Autodesk Fusion 360 part; units mm, degrees
note: some values were not read from the file. Set by a fixed rule: which sketch regions a step uses.
(part 3 of 4)
sketch "Boceto2" plane through (0, 0, 0) normal (0, 0, 1) x (1, 0, 0)
  line L0 (0, 0) -> (609.6, 0)
  line L1 (609.6, 0) -> (609.6, 800)
  line L2 (609.6, 800) -> (0, 800)
  line L3 (0, 800) -> (0, 0)
  line L4 (50, 750) -> (50, 50)
  line L5 (50, 50) -> (559.6, 50)
  line L6 (559.6, 50) -> (559.6, 750)
  line L7 (559.6, 750) -> (50, 750)
  line L8 (-347.6805, -725) -> (-296.8805, -725)
  line L9 (-347.6805, -725) -> (-296.8805, -725)
  line L10 (-525, -725) -> (-347.6805, -725)
  line L11 (-347.6805, -725) -> (-296.8805, -725)
  line L12 (-525, -725) -> (-347.6805, -725)
  line L13 (-347.6805, -725) -> (-373.0805, -725)
  line L14 (-525, -725) -> (-347.6805, -725)
  circle A0 centre (-525, -725) radius 228.1195
  line L15 (-347.6805, -725) -> (-373.0805, -725)
  circle A1 centre (-525, -725) radius 228.1195
  circle A2 centre (-373.0805, -725) radius 2.1
  line L16 (-347.6805, -725) -> (-296.8805, -725)
  circle A3 centre (-525, -725) radius 228.1195
  line L17 (-347.6805, -725) -> (-355.9463, -725)
  line L18 (-525, -725) -> (-525, -547.6805)
  line L19 (-525, -725) -> (-525, -547.6805)
  line L20 (-347.6805, -725) -> (-373.0805, -725)
  line L21 (-347.6805, -725) -> (-355.9463, -725)
  line L22 (-347.6805, -725) -> (-355.9463, -725)
  line L23 (-525, -725) -> (-525, -547.6805)
  line L24 (-525, -725) -> (-525, -547.6805)
  line L25 (-347.6805, -725) -> (-355.9463, -725)
  line L26 (-525, -725) -> (-347.6805, -725)
  line L27 (-525, -725) -> (-347.6805, -725)
  line L28 (-525, -725) -> (-347.6805, -725)
  line L29 (-347.6805, -725) -> (-355.9463, -725)
  line L30 (-347.6805, -725) -> (-296.8805, -725)
  line L31 (-347.6805, -725) -> (-296.8805, -725)
  line L32 (-347.6805, -725) -> (-355.9463, -725)
  line L33 (-347.6805, -725) -> (-296.8805, -725)
  line L34 (-347.6805, -725) -> (-296.8805, -725)
  line L35 (-525, -725) -> (-347.6805, -725)
  line L36 (-347.6805, -725) -> (-355.9463, -725)
  line L37 (-347.6805, -725) -> (-355.9463, -725)
  line L38 (-347.6805, -725) -> (-296.8805, -725)
  line L39 (-347.6805, -725) -> (-355.9463, -725)
  line L40 (-347.6805, -725) -> (-296.8805, -725)
  line L41 (-347.6805, -725) -> (-296.8805, -725)
  line L42 (-525, -725) -> (-347.6805, -725)
  line L43 (-347.6805, -725) -> (-373.0805, -725)
  line L44 (-347.6805, -725) -> (-373.0805, -725)
  line L45 (-525, -725) -> (-525, -547.6805)
  line L46 (-525, -725) -> (-525, -547.6805)
  line L47 (-347.6805, -725) -> (-373.0805, -725)
  circle A4 centre (-525, -725) radius 228.1195
  line L48 (-347.6805, -725) -> (-373.0805, -725)
  line L49 (-347.6805, -725) -> (-373.0805, -725)
  line L50 (-347.6805, -725) -> (-296.8805, -725)
  line L51 (-525, -725) -> (-525, -547.6805)
  line L52 (-347.6805, -725) -> (-373.0805, -725)
  line L53 (-347.6805, -725) -> (-296.8805, -725)
  circle A5 centre (-525, -725) radius 228.1195
  line L54 (-525, -725) -> (-525, -547.6805)
  line L55 (-347.6805, -725) -> (-355.9463, -725)
  line L56 (-347.6805, -725) -> (-355.9463, -725)
  line L57 (-525, -725) -> (-525, -547.6805)
  line L58 (-347.6805, -725) -> (-373.0805, -725)
  line L59 (-525, -725) -> (-525, -547.6805)
  line L60 (-347.6805, -725) -> (-355.9463, -725)
  line L61 (-347.6805, -725) -> (-355.9463, -725)
  line L62 (-525, -725) -> (-525, -547.6805)
  line L63 (-525, -725) -> (-347.6805, -725)
  line L64 (-525, -725) -> (-347.6805, -725)
  line L65 (-525, -725) -> (-347.6805, -725)
  line L66 (-525, -725) -> (-347.6805, -725)
  line L67 (-347.6805, -725) -> (-296.8805, -725)
  line L68 (-347.6805, -725) -> (-355.9463, -725)
  line L69 (-525, -725) -> (-347.6805, -725)
  line L70 (-347.6805, -725) -> (-296.8805, -725)
  line L71 (-347.6805, -725) -> (-355.9463, -725)
  circle A6 centre (-525, -725) radius 228.1195
  circle A7 centre (-525, -725) radius 228.1195
  circle A8 centre (-525, -725) radius 228.1195
  circle A9 centre (-525, -725) radius 228.1195
  line L72 (-525, -725) -> (-347.6805, -725)
  line L73 (-347.6805, -725) -> (-373.0805, -725)
  line L74 (-347.6805, -725) -> (-373.0805, -725)
  line L75 (-347.6805, -725) -> (-373.0805, -725)
  circle A10 centre (-525, -725) radius 228.1195
  line L76 (-347.6805, -725) -> (-373.0805, -725)
  circle A11 centre (-525, -725) radius 228.1195
  line L77 (-347.6805, -725) -> (-373.0805, -725)
  line L78 (-525, -725) -> (-347.6805, -725)
  circle A12 centre (-525, -725) radius 228.1195
  circle A13 centre (-373.0805, -725) radius 2.1
  circle A14 centre (-373.0805, -725) radius 2.1
  circle A15 centre (-373.0805, -725) radius 2.1
  line L79 (-347.6805, -725) -> (-373.0805, -725)
  line L80 (-347.6805, -725) -> (-355.9463, -725)
  line L81 (-525, -725) -> (-347.6805, -725)
  circle A16 centre (-525, -725) radius 228.1195
  circle A17 centre (-525, -725) radius 228.1195
  line L82 (-347.6805, -725) -> (-296.8805, -725)
  circle A18 centre (-525, -725) radius 228.1195
  line L83 (-525, -547.6805) -> (-525, -573.0805)
  circle A19 centre (-525, -573.0805) radius 2.1
  line L84 (-525, -547.6805) -> (-525, -573.0805)
  circle A20 centre (-525, -573.0805) radius 2.1
  line L85 (-525, -547.6805) -> (-525, -573.0805)
  line L86 (-525, -547.6805) -> (-525, -573.0805)
  line L87 (-525, -725) -> (-525, -547.6805)
  circle A21 centre (-525, -573.0805) radius 2.1
  line L88 (-525, -547.6805) -> (-525, -573.0805)
  line L89 (-525, -547.6805) -> (-525, -573.0805)
  line L90 (-525, -902.3195) -> (-525, -876.9195)
  line L91 (-525, -725) -> (-702.3195, -725)
  line L92 (-525, -725) -> (-702.3195, -725)
  line L93 (-525, -902.3195) -> (-525, -876.9195)
  line L94 (-525, -725) -> (-525, -547.6805)
  circle A22 centre (-525, -876.9195) radius 2.1
  circle A23 centre (-525, -573.0805) radius 2.1
  circle A24 centre (-525, -573.0805) radius 2.1
  line L95 (-525, -547.6805) -> (-525, -573.0805)
  line L96 (-525, -902.3195) -> (-525, -876.9195)
  line L97 (-525, -547.6805) -> (-525, -573.0805)
  line L98 (-525, -547.6805) -> (-525, -573.0805)
  circle A25 centre (-525, -573.0805) radius 2.1
  line L99 (-525, -725) -> (-702.3195, -725)
  line L100 (-525, -725) -> (-702.3195, -725)
  line L101 (-525, -547.6805) -> (-525, -573.0805)
  line L102 (-525, -725) -> (-702.3195, -725)
  circle A26 centre (-525, -573.0805) radius 2.1
  line L103 (-525, -547.6805) -> (-525, -573.0805)
  line L104 (-525, -547.6805) -> (-525, -573.0805)
  line L105 (-525, -725) -> (-525, -902.3195)
  circle A27 centre (-525, -876.9195) radius 2.1
  line L106 (-525, -725) -> (-525, -902.3195)
  line L107 (-525, -547.6805) -> (-525, -573.0805)
  circle A28 centre (-525, -876.9195) radius 2.1
  line L108 (-525, -902.3195) -> (-525, -876.9195)
  circle A29 centre (-525, -573.0805) radius 2.1
  circle A30 centre (-525, -573.0805) radius 2.1
  line L109 (-525, -725) -> (-525, -547.6805)
  line L110 (-525, -725) -> (-525, -547.6805)
  circle A31 centre (-525, -876.9195) radius 2.1
  circle A32 centre (-525, -573.0805) radius 2.1
  line L111 (-525, -902.3195) -> (-525, -876.9195)
  line L112 (-525, -725) -> (-525, -902.3195)
  line L113 (-525, -725) -> (-525, -902.3195)
  line L114 (-525, -902.3195) -> (-525, -876.9195)
  line L115 (-525, -725) -> (-525, -902.3195)
  line L116 (-525, -725) -> (-525, -547.6805)
  line L117 (-525, -547.6805) -> (-525, -573.0805)
  line L118 (-525, -725) -> (-702.3195, -725)
  line L119 (-525, -725) -> (-702.3195, -725)
  circle A33 centre (-525, -573.0805) radius 2.1
  line L120 (-525, -902.3195) -> (-525, -876.9195)
  line L121 (-525, -547.6805) -> (-525, -573.0805)
  circle A34 centre (-525, -573.0805) radius 2.1
  circle A35 centre (-525, -573.0805) radius 2.1
  line L122 (-525, -902.3195) -> (-525, -876.9195)
  line L123 (-525, -725) -> (-525, -902.3195)
  circle A36 centre (-525, -573.0805) radius 2.1
  line L124 (-525, -547.6805) -> (-525, -573.0805)
  line L125 (-525, -725) -> (-702.3195, -725)
  circle A37 centre (-525, -573.0805) radius 2.1
  circle A38 centre (-525, -573.0805) radius 2.1
  circle A39 centre (-525, -876.9195) radius 2.1
  circle A40 centre (-676.9195, -725) radius 2.1
  line L126 (-525, -725) -> (-702.3195, -725)
  circle A41 centre (-676.9195, -725) radius 2.1
  circle A42 centre (-676.9195, -725) radius 2.1
  line L127 (-702.3195, -725) -> (-676.9195, -725)
  line L128 (-525, -902.3195) -> (-525, -876.9195)
  circle A43 centre (-676.9195, -725) radius 2.1
  circle A44 centre (-676.9195, -725) radius 2.1
  line L129 (-525, -902.3195) -> (-525, -876.9195)
  line L130 (-525, -725) -> (-525, -902.3195)
  circle A45 centre (-525, -876.9195) radius 2.1
  line L131 (-525, -725) -> (-702.3195, -725)
  circle A46 centre (-525, -876.9195) radius 2.1
  line L132 (-525, -725) -> (-525, -902.3195)
  line L133 (-525, -725) -> (-525, -902.3195)
  line L134 (-525, -725) -> (-525, -902.3195)
  circle A47 centre (-525, -876.9195) radius 2.1
  line L135 (-525, -725) -> (-702.3195, -725)
  line L136 (-525, -725) -> (-702.3195, -725)
  line L137 (-702.3195, -725) -> (-676.9195, -725)
  line L138 (-702.3195, -725) -> (-676.9195, -725)
  circle A48 centre (-676.9195, -725) radius 2.1
  line L139 (-525, -902.3195) -> (-525, -876.9195)
  circle A49 centre (-525, -876.9195) radius 2.1
  line L140 (-525, -725) -> (-525, -902.3195)
  line L141 (-525, -725) -> (-525, -902.3195)
  circle A50 centre (-525, -876.9195) radius 2.1
  circle A51 centre (-525, -876.9195) radius 2.1
  line L142 (-525, -725) -> (-702.3195, -725)
  line L143 (-525, -902.3195) -> (-525, -876.9195)
  line L144 (-525, -725) -> (-702.3195, -725)
  line L145 (-525, -725) -> (-702.3195, -725)
  line L146 (-525, -902.3195) -> (-525, -876.9195)
  circle A52 centre (-525, -876.9195) radius 2.1
  circle A53 centre (-525, -876.9195) radius 2.1
  line L147 (-525, -725) -> (-525, -902.3195)
  line L148 (-525, -902.3195) -> (-525, -876.9195)
  line L149 (-525, -902.3195) -> (-525, -876.9195)
  circle A54 centre (-676.9195, -725) radius 2.1
  line L150 (-525, -725) -> (-525, -902.3195)
  circle A55 centre (-676.9195, -725) radius 2.1
  line L151 (-525, -725) -> (-702.3195, -725)
  line L152 (-525, -902.3195) -> (-525, -876.9195)
  circle A56 centre (-676.9195, -725) radius 2.1
  line L153 (-525, -725) -> (-525, -902.3195)
  line L154 (-525, -725) -> (-525, -902.3195)
  circle A57 centre (-525, -876.9195) radius 2.1
  circle A58 centre (-525, -876.9195) radius 2.1
  circle A59 centre (-525, -876.9195) radius 2.1
  circle A60 centre (-676.9195, -725) radius 2.1
  line L155 (-702.3195, -725) -> (-676.9195, -725)
  line L156 (-702.3195, -725) -> (-676.9195, -725)
  line L157 (-702.3195, -725) -> (-676.9195, -725)
  line L158 (-702.3195, -725) -> (-676.9195, -725)
  line L159 (-702.3195, -725) -> (-676.9195, -725)
  circle A61 centre (-676.9195, -725) radius 2.1
  line L160 (-702.3195, -725) -> (-676.9195, -725)
  line L161 (-702.3195, -725) -> (-676.9195, -725)
  circle A62 centre (-676.9195, -725) radius 2.1
  line L162 (-702.3195, -725) -> (-676.9195, -725)
  line L163 (-702.3195, -725) -> (-676.9195, -725)
  circle A63 centre (-676.9195, -725) radius 2.1
  circle A64 centre (-676.9195, -725) radius 2.1
  line L164 (-702.3195, -725) -> (-676.9195, -725)
  line L165 (-702.3195, -725) -> (-676.9195, -725)
  line L166 (-702.3195, -725) -> (-676.9195, -725)
  circle A65 centre (-676.9195, -725) radius 2.1
  circle A66 centre (-676.9195, -725) radius 2.1
  line L167 (-702.3195, -725) -> (-676.9195, -725)
  circle A67 centre (-373.0805, -725) radius 2.1
  circle A68 centre (-373.0805, -725) radius 2.1
  circle A69 centre (-373.0805, -725) radius 2.1
  circle A70 centre (-525, -725) radius 228.1195
  circle A71 centre (-373.0805, -725) radius 2.1
  circle A72 centre (-373.0805, -725) radius 2.1
  circle A73 centre (-373.0805, -725) radius 2.1
  circle A74 centre (-373.0805, -725) radius 2.1
  circle A75 centre (-373.0805, -725) radius 2.1
  circle A76 centre (-373.0805, -725) radius 2.1
  circle A77 centre (-373.0805, -725) radius 2.1
  circle A78 centre (-373.0805, -725) radius 2.1
  circle A79 centre (-373.0805, -725) radius 2.1
  circle A80 centre (-525, -725) radius 228.1195
  circle A81 centre (304.8, 400) radius 228.1195
  circle A82 centre (304.8, 400) radius 238.1195
  dimension "d627" = 609.6
  dimension "d628" = 800
  dimension "d736" = -50
  dimension "d737" = 177.3195
  dimension "d738" = 177.3195
  dimension "d739" = 177.3195
  dimension "d740" = 177.3195
  dimension "d741" = 25.4
  dimension "d742" = 25.4
  dimension "d743" = 25.4
  dimension "d744" = 25.4
  dimension "d745" = 4.2
  dimension "d746" = 4.2
  dimension "d747" = 4.2
  dimension "d748" = 4.2
  dimension "d749" = 50.8
  dimension "d750" = 177.3195
  dimension "d751" = 177.3195
  dimension "d752" = 177.3195
  dimension "d753" = 177.3195
  dimension "d754" = 25.4
  dimension "d755" = 25.4
  dimension "d756" = 25.4
  dimension "d757" = 25.4
  dimension "d758" = 4.2
  dimension "d759" = 4.2
  dimension "d760" = 4.2
  dimension "d761" = 4.2
  dimension "d762" = 50.8
  dimension "d763" = 177.3195
  dimension "d764" = 177.3195
  dimension "d765" = 177.3195
  dimension "d766" = 177.3195
  dimension "d767" = 25.4
  dimension "d768" = 25.4
  dimension "d769" = 25.4
  dimension "d770" = 25.4
  dimension "d771" = 4.2
  dimension "d772" = 4.2
  dimension "d773" = 4.2
  dimension "d774" = 4.2
  dimension "d775" = 50.8
  dimension "d776" = 177.3195
  dimension "d777" = 177.3195
  dimension "d778" = 177.3195
  dimension "d779" = 177.3195
  dimension "d780" = 25.4
  dimension "d781" = 25.4
  dimension "d782" = 25.4
  dimension "d783" = 25.4
  dimension "d784" = 4.2
  dimension "d785" = 4.2
  dimension "d786" = 4.2
  dimension "d787" = 4.2
  dimension "d788" = 50.8
  dimension "d789" = 177.3195
  dimension "d790" = 177.3195
  dimension "d791" = 177.3195
  dimension "d792" = 177.3195
  dimension "d793" = 25.4
  dimension "d794" = 25.4
  dimension "d795" = 25.4
  dimension "d796" = 25.4
  dimension "d797" = 4.2
  dimension "d798" = 4.2
  dimension "d799" = 4.2
  dimension "d800" = 4.2
  dimension "d801" = 50.8
  dimension "d802" = 177.3195
  dimension "d803" = 177.3195
  dimension "d804" = 177.3195
  dimension "d805" = 177.3195
  dimension "d806" = 25.4
  dimension "d807" = 25.4
  dimension "d808" = 25.4
  dimension "d809" = 25.4
  dimension "d810" = 4.2
  dimension "d811" = 4.2
  dimension "d812" = 4.2
  dimension "d813" = 4.2
  dimension "d814" = 50.8
  dimension "d815" = 177.3195
  dimension "d816" = 177.3195
  dimension "d817" = 177.3195
  dimension "d818" = 177.3195
  dimension "d819" = 25.4
  dimension "d820" = 25.4
  dimension "d821" = 25.4
  dimension "d822" = 25.4
  dimension "d823" = 4.2
  dimension "d824" = 4.2
  dimension "d825" = 4.2
  dimension "d826" = 4.2
  dimension "d827" = 50.8
  dimension "d828" = 177.3195
  dimension "d829" = 177.3195
  dimension "d830" = 177.3195
  dimension "d831" = 177.3195
  dimension "d832" = 25.4
  dimension "d833" = 25.4
  dimension "d834" = 25.4
  dimension "d835" = 25.4
  dimension "d836" = 4.2
  dimension "d837" = 4.2
  dimension "d838" = 4.2
  dimension "d839" = 4.2
  dimension "d840" = 50.8
  dimension "d841" = 177.3195
  dimension "d842" = 177.3195
  dimension "d843" = 177.3195
  dimension "d844" = 177.3195
  dimension "d845" = 25.4
  dimension "d846" = 25.4
  dimension "d847" = 25.4
  dimension "d848" = 25.4
  dimension "d849" = 4.2
  dimension "d850" = 4.2
  dimension "d851" = 4.2
  dimension "d852" = 4.2
  dimension "d853" = 50.8
  dimension "d854" = 177.3195
  dimension "d855" = 177.3195
  dimension "d856" = 177.3195
  dimension "d857" = 177.3195
  dimension "d858" = 25.4
  dimension "d859" = 25.4
  dimension "d860" = 25.4
  dimension "d861" = 25.4
  dimension "d862" = 4.2
  dimension "d863" = 4.2
  dimension "d864" = 4.2
  dimension "d865" = 4.2
  dimension "d866" = 50.8
  dimension "d867" = 177.3195
  dimension "d868" = 177.3195
  dimension "d869" = 177.3195
  dimension "d870" = 177.3195
  dimension "d871" = 25.4
  dimension "d872" = 25.4
  dimension "d873" = 25.4
  dimension "d874" = 25.4
  dimension "d875" = 4.2
  dimension "d876" = 4.2
  dimension "d877" = 4.2
  dimension "d878" = 4.2
  dimension "d879" = 50.8
  dimension "d880" = 177.3195
  dimension "d881" = 177.3195
  dimension "d882" = 177.3195
  dimension "d883" = 177.3195
  dimension "d884" = 25.4
  dimension "d885" = 25.4
  dimension "d886" = 25.4
  dimension "d887" = 25.4
  dimension "d888" = 4.2
  dimension "d889" = 4.2
  dimension "d890" = 4.2
  dimension "d891" = 4.2
  dimension "d892" = 50.8
  dimension "d893" = 177.3195
  dimension "d894" = 177.3195
  dimension "d895" = 177.3195
  dimension "d896" = 177.3195
  dimension "d897" = 25.4
  dimension "d898" = 25.4
  dimension "d904" = 25.4
  dimension "d905" = 25.4
  dimension "d906" = 4.2
  dimension "d912" = 4.2
  dimension "d916" = 4.2
  dimension "d917" = 4.2
  dimension "d918" = 50.8
  dimension "d921" = 177.3195
  dimension "d922" = 177.3195
  dimension "d924" = 177.3195
  dimension "d925" = 177.3195
  dimension "d926" = 25.4
  dimension "d929" = 25.4
  dimension "d930" = 25.4
  dimension "d931" = 25.4
  dimension "d932" = 4.2
  dimension "d934" = 4.2
  dimension "d935" = 4.2
  dimension "d936" = 4.2
  dimension "d940" = 50.8
  dimension "d944" = 177.3195
  dimension "d945" = 177.3195
  dimension "d946" = 177.3195
  dimension "d947" = 177.3195
  dimension "d948" = 25.4
  dimension "d951" = 25.4
  dimension "d952" = 25.4
  dimension "d953" = 25.4
  dimension "d954" = 4.2
  dimension "d955" = 4.2
  dimension "d956" = 4.2
  dimension "d957" = 4.2
  dimension "d958" = 50.8
  dimension "d959" = 177.3195
  dimension "d960" = 177.3195
  dimension "d961" = 177.3195
  dimension "d962" = 177.3195
  dimension "d963" = 25.4
  dimension "d964" = 25.4
  dimension "d965" = 25.4
  dimension "d966" = 25.4
  dimension "d967" = 4.2
  dimension "d968" = 4.2
  dimension "d969" = 4.2
  dimension "d970" = 4.2
  dimension "d971" = 50.8
  dimension "d972" = 456.2391
  dimension "d973" = 456.239
  dimension "d974" = 10
  constraint horizontal L0
  constraint vertical L1
  constraint horizontal L2
  constraint vertical L3
  constraint coincident L0.start L3.end
  constraint vertical L140
  constraint perpendicular L81 L140
  constraint perpendicular L100 L140
  constraint perpendicular L46 L81
  constraint coincident L17.end L81
  constraint parallel L76 L81
  constraint parallel L46 L88
  constraint parallel L100 L157
  constraint parallel L140 L143
  constraint coincident L13.end L15.end
  constraint coincident L83.end A19.centre
  constraint coincident A40.centre A41.centre
  constraint coincident L90.end L93.end
  constraint parallel L70 L81
  constraint coincident L10.start L12.start
  constraint coincident L8.end A6
  constraint vertical L123
  constraint perpendicular L78 L123
  constraint perpendicular L119 L123
  constraint perpendicular L78 L116
  constraint coincident L17.end L78
  constraint parallel L43 L78
  constraint parallel L103 L116
  constraint parallel L119 L160
  constraint parallel L123 L149
  constraint parallel L11 L78
  constraint coincident L8.end A0
  constraint vertical L106
  constraint perpendicular L10 L106
  constraint perpendicular L91 L106
  constraint perpendicular L10 L24
  constraint coincident L17.end L10
  constraint parallel L10 L48
  constraint parallel L24 L101
  constraint parallel L91 L158
  constraint parallel L106 L152
  constraint parallel L10 L38
  constraint coincident L8.end A10
  constraint vertical L147
  constraint perpendicular L66 L147
  constraint perpendicular L118 L147
  constraint perpendicular L45 L66
  constraint coincident L17.end L66
  constraint parallel L13 L66
  constraint parallel L45 L83
  constraint parallel L118 L164
  constraint parallel L120 L147
  constraint parallel L53 L66
  constraint coincident L8.end A7
  constraint vertical L154
  constraint perpendicular L63 L154
  constraint perpendicular L136 L154
  constraint perpendicular L18 L63
  constraint coincident L17.end L63
  constraint parallel L49 L63
  constraint parallel L18 L89
  constraint parallel L136 L137
  constraint parallel L111 L154
  constraint parallel L50 L63
  constraint coincident L8.end A1
  constraint vertical L141
  constraint perpendicular L72 L141
  constraint perpendicular L141 L142
  constraint perpendicular L19 L72
  constraint coincident L17.end L72
  constraint parallel L58 L72
  constraint parallel L19 L104
  constraint parallel L142 L162
  constraint parallel L129 L141
  constraint parallel L8 L72
  constraint coincident L8.end A9
  constraint vertical L115
  constraint perpendicular L28 L115
  constraint perpendicular L92 L115
  constraint perpendicular L28 L110
  constraint coincident L17.end L28
  constraint parallel L28 L77
  constraint parallel L85 L110
  constraint parallel L92 L155
  constraint parallel L108 L115
  constraint parallel L28 L40
  constraint coincident L8.end A11
  constraint vertical L153
  constraint perpendicular L65 L153
  constraint perpendicular L144 L153
  constraint perpendicular L62 L65
  constraint coincident L17.end L65
  constraint parallel L20 L65
  constraint parallel L62 L95
  constraint parallel L144 L165
  constraint parallel L96 L153
  constraint parallel L65 L67
  constraint coincident L8.end A4
  constraint vertical L132
  constraint perpendicular L12 L132
  constraint perpendicular L126 L132
  constraint perpendicular L12 L23
  constraint coincident L17.end L12
  constraint parallel L12 L75
  constraint parallel L23 L124
  constraint parallel L126 L163
  constraint parallel L114 L132
  constraint parallel L12 L82
  constraint coincident L8.end A12
  constraint vertical L112
  constraint perpendicular L35 L112
  constraint perpendicular L112 L151
  constraint perpendicular L35 L109
  constraint coincident L17.end L35
  constraint parallel L35 L79
  constraint parallel L109 L117
  constraint parallel L151 L159
  constraint parallel L112 L139
  constraint parallel L16 L35
  constraint coincident L8.end A70
  constraint vertical L113
  constraint perpendicular L64 L113
  constraint perpendicular L113 L125
  constraint perpendicular L64 L87
  constraint coincident L17.end L64
  constraint parallel L64 L74
  constraint parallel L86 L87
  constraint parallel L125 L166
  constraint parallel L113 L148
  constraint parallel L30 L64
  constraint coincident L8.end A5
  constraint vertical L133
  constraint perpendicular L27 L133
  constraint perpendicular L99 L133
  constraint perpendicular L27 L54
  constraint coincident L17.end L27
  constraint parallel L15 L27
  constraint parallel L54 L98
  constraint parallel L99 L127
  constraint parallel L93 L133
  constraint parallel L27 L34
  constraint coincident L8.end A17
  constraint vertical L130
  constraint perpendicular L14 L130
  constraint perpendicular L130 L131
  constraint perpendicular L14 L94
  constraint coincident L17.end L14
  constraint parallel L14 L52
  constraint parallel L84 L94
  constraint parallel L131 L161
  constraint parallel L122 L130
  constraint parallel L9 L14
  constraint coincident L8.end A8
  constraint vertical L105
  constraint perpendicular L42 L105
  constraint perpendicular L102 L105
  constraint perpendicular L42 L59
  constraint coincident L17.end L42
  constraint parallel L42 L47
  constraint parallel L59 L107
  constraint parallel L102 L156
  constraint parallel L105 L146
  constraint parallel L33 L42
  constraint coincident L8.end A16
  constraint vertical L150
  constraint perpendicular L26 L150
  constraint perpendicular L135 L150
  constraint perpendicular L26 L57
  constraint coincident L17.end L26
  constraint parallel L26 L73
  constraint parallel L57 L97
  constraint parallel L135 L138
  constraint parallel L128 L150
  constraint parallel L26 L31
  constraint coincident L8.end A3
  constraint vertical L134
  constraint perpendicular L69 L134
  constraint perpendicular L134 L145
  constraint perpendicular L51 L69
  constraint coincident L17.end L69
  constraint parallel L44 L69
  constraint parallel L51 L121
  constraint parallel L145 L167
  constraint parallel L90 L134
  constraint parallel L41 L69
  constraint coincident L8.end A18
  measures "d627" distance of L0.start L0.end
  measures "d628" distance of L0.start L2.end
  measures "d737" distance of L10.start L90.start
  measures "d738" distance of L10.start L8.start
  measures "d739" distance of L10.start L91.end
  measures "d740" distance of L10.start L18.end
  measures "d741" distance of L8.start L13.end
  measures "d742" distance of L18.end L83.end
  measures "d743" distance of L91.end A40.centre
  measures "d744" distance of L90.end L90.start
  measures "d745" diameter of A13
  measures "d746" diameter of A37
  measures "d747" diameter of A54
  measures "d748" diameter of A51
  measures "d749" distance of L8.start L8.end
  measures "d750" distance of L90.start L10.start
  measures "d751" distance of L10.start L8.start
  measures "d752" distance of L91.end L10.start
  measures "d753" distance of L18.end L10.start
  measures "d754" distance of L13.end L8.start
  measures "d755" distance of L83.end L18.end
  measures "d756" distance of L91.end A40.centre
  measures "d757" distance of L90.start L90.end
  measures "d758" diameter of A71
  measures "d759" diameter of A30
  measures "d760" diameter of A56
  measures "d761" diameter of A31
  measures "d762" distance of L8.end L8.start
  measures "d763" distance of L10.start L90.start
  measures "d764" distance of L10.start L8.start
  measures "d765" distance of L10.start L91.end
  measures "d766" distance of L10.start L18.end
  measures "d767" distance of L8.start L13.end
  measures "d768" distance of L83.end L18.end
  measures "d769" distance of L91.end A40.centre
  measures "d770" distance of L90.end L90.start
  measures "d771" diameter of A79
  measures "d772" diameter of A19
  measures "d773" diameter of A65
  measures "d774" diameter of A50
  measures "d775" distance of L8.end L8.start
  measures "d776" distance of L10.start L90.start
  measures "d777" distance of L10.start L8.start
  measures "d778" distance of L91.end L10.start
  measures "d779" distance of L18.end L10.start
  measures "d780" distance of L13.end L8.start
  measures "d781" distance of L18.end L83.end
  measures "d782" distance of L91.end A40.centre
  measures "d783" distance of L90.end L90.start
  measures "d784" diameter of A14
  measures "d785" diameter of A33
  measures "d786" diameter of A61
  measures "d787" diameter of A22
  measures "d788" distance of L8.end L8.start
  measures "d789" distance of L90.start L10.start
  measures "d790" distance of L8.start L10.start
  measures "d791" distance of L91.end L10.start
  measures "d792" distance of L18.end L10.start
  measures "d793" distance of L13.end L8.start
  measures "d794" distance of L18.end L83.end
  measures "d795" distance of A40.centre L91.end
  measures "d796" distance of L90.start L90.end
  measures "d797" diameter of A67
  measures "d798" diameter of A38
  measures "d799" diameter of A55
  measures "d800" diameter of A46
  measures "d801" distance of L8.start L8.end
  measures "d802" distance of L90.start L10.start
  measures "d803" distance of L8.start L10.start
  measures "d804" distance of L91.end L10.start
  measures "d805" distance of L18.end L10.start
  measures "d806" distance of L13.end L8.start
  measures "d807" distance of L83.end L18.end
  measures "d808" distance of A40.centre L91.end
  measures "d809" distance of L90.end L90.start
  measures "d810" diameter of A72
  measures "d811" diameter of A25
  measures "d812" diameter of A60
  measures "d813" diameter of A47
  measures "d814" distance of L8.end L8.start
  measures "d815" distance of L10.start L90.start
  measures "d816" distance of L10.start L8.start
  measures "d817" distance of L10.start L91.end
  measures "d818" distance of L10.start L18.end
  measures "d819" distance of L13.end L8.start
  measures "d820" distance of L18.end L83.end
  measures "d821" distance of A40.centre L91.end
  measures "d822" distance of L90.start L90.end
  measures "d823" diameter of A15
  measures "d824" diameter of A23
  measures "d825" diameter of A43
  measures "d826" diameter of A58
  measures "d827" distance of L8.end L8.start
  measures "d828" distance of L90.start L10.start
  measures "d829" distance of L8.start L10.start
  measures "d830" distance of L91.end L10.start
  measures "d831" distance of L18.end L10.start
  measures "d832" distance of L8.start L13.end
  measures "d833" distance of L18.end L83.end
  measures "d834" distance of A40.centre L91.end
  measures "d835" distance of L90.start L90.end
  measures "d836" diameter of A69
  measures "d837" diameter of A35
  measures "d838" diameter of A44
  measures "d839" diameter of A39
  measures "d840" distance of L8.start L8.end
  measures "d841" distance of L90.start L10.start
  measures "d842" distance of L10.start L8.start
  measures "d843" distance of L10.start L91.end
  measures "d844" distance of L18.end L10.start
  measures "d845" distance of L13.end L8.start
  measures "d846" distance of L83.end L18.end
  measures "d847" distance of A40.centre L91.end
  measures "d848" distance of L90.start L90.end
  measures "d849" diameter of A77
  measures "d850" diameter of A21
  measures "d851" diameter of A42
  measures "d852" diameter of A45
  measures "d853" distance of L8.end L8.start
  measures "d854" distance of L90.start L10.start
  measures "d855" distance of L10.start L8.start
  measures "d856" distance of L91.end L10.start
  measures "d857" distance of L10.start L18.end
  measures "d858" distance of L13.end L8.start
  measures "d859" distance of L83.end L18.end
  measures "d860" distance of L91.end A40.centre
  measures "d861" distance of L90.start L90.end
  measures "d862" diameter of A2
  measures "d863" diameter of A29
  measures "d864" diameter of A48
  measures "d865" diameter of A59
  measures "d866" distance of L8.end L8.start
  measures "d867" distance of L10.start L90.start
  measures "d868" distance of L10.start L8.start
  measures "d869" distance of L10.start L91.end
  measures "d870" distance of L10.start L18.end
  measures "d871" distance of L8.start L13.end
  measures "d872" distance of L18.end L83.end
  measures "d873" distance of A40.centre L91.end
  measures "d874" distance of L90.end L90.start
  measures "d875" diameter of A78
  measures "d876" diameter of A24
  measures "d877" diameter of A40
  measures "d878" diameter of A57
  measures "d879" distance of L8.end L8.start
  measures "d880" distance of L10.start L90.start
  measures "d881" distance of L10.start L8.start
  measures "d882" distance of L91.end L10.start
  measures "d883" distance of L18.end L10.start
  measures "d884" distance of L13.end L8.start
  measures "d885" distance of L18.end L83.end
  measures "d886" distance of L91.end A40.centre
  measures "d887" distance of L90.end L90.start
  measures "d888" diameter of A76
  measures "d889" diameter of A36
  measures "d890" diameter of A66
  measures "d891" diameter of A49
  measures "d892" distance of L8.end L8.start
  measures "d893" distance of L90.start L10.start
  measures "d894" distance of L10.start L8.start
  measures "d895" distance of L10.start L91.end
  measures "d896" distance of L18.end L10.start
  measures "d897" distance of L8.start L13.end
  measures "d898" distance of L18.end L83.end
  measures "d904" distance of L91.end A40.centre
  measures "d905" distance of L90.start L90.end
  measures "d906" diameter of A73
  measures "d912" diameter of A20
  measures "d916" diameter of A64
  measures "d917" diameter of A27
  measures "d918" distance of L8.end L8.start
  measures "d921" distance of L10.start L90.start
  measures "d922" distance of L10.start L8.start
  measures "d924" distance of L91.end L10.start
  measures "d925" distance of L18.end L10.start
  measures "d926" distance of L8.start L13.end
  measures "d929" distance of L18.end L83.end
  measures "d930" distance of L91.end A40.centre
  measures "d931" distance of L90.end L90.start
  measures "d932" diameter of A74
  measures "d934" diameter of A26
  measures "d935" diameter of A41
  measures "d936" diameter of A28
  measures "d940" distance of L8.start L8.end
  measures "d944" distance of L10.start L90.start
  measures "d945" distance of L8.start L10.start
  measures "d946" distance of L91.end L10.start
  measures "d947" distance of L10.start L18.end
  measures "d948" distance of L8.start L13.end
  measures "d951" distance of L18.end L83.end
  measures "d952" distance of A40.centre L91.end
  measures "d953" distance of L90.end L90.start
  measures "d954" diameter of A75
  measures "d955" diameter of A34
  measures "d956" diameter of A62
  measures "d957" diameter of A52
  measures "d958" distance of L8.start L8.end
  measures "d959" distance of L10.start L90.start
  measures "d960" distance of L10.start L8.start
  measures "d961" distance of L10.start L91.end
  measures "d962" distance of L10.start L18.end
  measures "d963" distance of L13.end L8.start
  measures "d964" distance of L18.end L83.end
  measures "d965" distance of L91.end A40.centre
  measures "d966" distance of L90.end L90.start
  measures "d967" diameter of A68
  measures "d968" diameter of A32
  measures "d969" diameter of A63
  measures "d970" diameter of A53
  measures "d971" distance of L8.end L8.start
  measures "d972" diameter of A80
  measures "d973" diameter of A81
extrude "Extruir1" add sketch "Boceto2" along normal blind 105 contours L0 L1 L2 L3
extrude "Extruir2" add sketch "Boceto2" along normal blind 50 contours L4 L5 L6 L7 | A81 | A82
sketch "Boceto3" plane through (0, 0, 50) normal (0, 0, 1) x (-1, 0, 0)
  line L0 (-559.6, -750) -> (-50, -750)
  line L1 (-50, -750) -> (-50, -50)
  line L2 (-50, -50) -> (-559.6, -50)
  line L3 (-559.6, -50) -> (-559.6, -750)
  line L4 (-50, -750) -> (-559.6, -750)
  line L5 (-559.6, -750) -> (-559.6, -50)
  line L6 (-50, -50) -> (-50, -750)
  line L7 (-559.6, -50) -> (-50, -50)
  circle A0 centre (-304.8, -400) radius 228.1195
  dimension "d984" = 456.239
  measures "d984" diameter of A0
extrude "Extruir4" add sketch "Boceto3" along normal blind 16
sketch "Boceto4" plane through (0, 0, 66) normal (0, 0, 1) x (-1, 0, 0)
  circle A0 centre (-304.8, -400) radius 228.1195
  line L0 (-559.6, -50) -> (-559.6, -750)
  line L1 (-559.6, -750) -> (-50, -750)
  line L2 (-50, -750) -> (-50, -50)
  line L3 (-50, -50) -> (-559.6, -50)
  circle A1 centre (-304.8, -400) radius 228.1195
  circle A2 centre (-304.8, -400) radius 228.1195
  circle A3 centre (-304.8, -400) radius 238.1195
  dimension "d987" = 10
  constraint concentric A1 A2
extrude "Extruir5" add sketch "Boceto4" along normal blind 20 contours L0 L1 L2 L3
fillet "Empalme1" radius 225 1 edges at (526.8053, 486.1077, 66)
sketch "Boceto5" plane through (609.6, 0, 0) normal (1, 0, 0) x (0, 1, 0)
  line L0 (0, 0) -> (800, 0)
  line L1 (800, 0) -> (800, 105)
  line L2 (800, 105) -> (0, 105)
  line L3 (0, 105) -> (0, 0)
  line L4 (0, 105) -> (800, 105)
  line L5 (0, 0) -> (0, 105)
  line L6 (0, 0) -> (800, 0)
  line L7 (800, 0) -> (800, 105)
  line L8 (0, 0) -> (800, 0)
  line L9 (800, 0) -> (800, 50)
  line L10 (800, 50) -> (0, 50)
  line L11 (0, 50) -> (0, 0)
  line L12 (0, 50) -> (0, 25)
  line L13 (0, 50) -> (100, 50)
  line L14 (0, 15) -> (0, 50)
  line L15 (0, 0) -> (140, 0)
  line L16 (140, 0) -> (140, 25)
  line L17 (140, 25) -> (0, 25)
  line L18 (0, 25) -> (0, 0)
  line L19 (140, 25) -> (140, 35)
  line L20 (140, 35) -> (300, 35)
  line L21 (300, 35) -> (300, 15)
  line L22 (300, 15) -> (140, 15)
  line L23 (140, 15) -> (140, 35)
  line L24 (800, 50) -> (660, 50)
  line L25 (660, 50) -> (660, 25)
  line L26 (660, 25) -> (800, 25)
  line L27 (800, 25) -> (800, 50)
  line L28 (660, 25) -> (660, 35)
  line L29 (660, 35) -> (500, 35)
  line L30 (500, 35) -> (500, 15)
  line L31 (500, 15) -> (660, 15)
  line L32 (660, 15) -> (660, 35)
  line L33 (300, 25) -> (500, 25)
  circle A0 centre (400, 25) radius 10
  circle A1 centre (400, 25) radius 19
  line L34 (659, 44) -> (501, 44)
  line L35 (491, 34) -> (491, 16)
  line L36 (501, 6) -> (659, 6)
  line L37 (669, 16) -> (669, 34)
  line L38 (143, 42) -> (297, 42)
  line L39 (307, 32) -> (307, 18)
  line L40 (297, 8) -> (143, 8)
  line L41 (133, 18) -> (133, 32)
  arc A2 (143, 42) -> (133, 32) centre (143, 32) ccw
  arc A3 (133, 18) -> (143, 8) centre (143, 18) ccw
  arc A4 (307, 32) -> (297, 42) centre (297, 32) ccw
  arc A5 (297, 8) -> (307, 18) centre (297, 18) ccw
  arc A6 (501, 44) -> (491, 34) centre (501, 34) ccw
  arc A7 (491, 16) -> (501, 6) centre (501, 16) ccw
  arc A8 (659, 6) -> (669, 16) centre (659, 16) ccw
  arc A9 (669, 34) -> (659, 44) centre (659, 34) ccw
  dimension "d992" = 800
  dimension "d993" = 50
  dimension "d997" = 140
  dimension "d998" = 10
  dimension "d999" = 160
  dimension "d1000" = 20
  dimension "d1001" = 140
  dimension "d1002" = 10
  dimension "d1003" = 160
  dimension "d1004" = 20
  dimension "d1005" = 9
  dimension "d1008" = 10
  dimension "d1009" = 10
  constraint horizontal L8
  constraint vertical L9
  constraint horizontal L10
  constraint vertical L11
  constraint coincident L0.start L3.end
  constraint midpoint L11 L12.end
  constraint horizontal L13
  constraint vertical L14
  constraint horizontal L15
  constraint vertical L16
  constraint horizontal L17
  constraint vertical L18
  constraint perpendicular L10 L19
  constraint horizontal L20
  constraint vertical L21
  constraint horizontal L22
  constraint vertical L23
  constraint horizontal L24
  constraint vertical L25
  constraint horizontal L26
  constraint vertical L27
  constraint perpendicular L26 L28
  constraint horizontal L29
  constraint vertical L30
  constraint horizontal L31
  constraint vertical L32
  constraint midpoint L21 L33.start
  constraint midpoint L30 L33.end
  constraint perpendicular L30 L33
  constraint midpoint L33 A0.centre
  constraint tangent L38 A2
  constraint tangent L41 A2
  constraint tangent L40 A3
  constraint tangent L41 A3
  constraint equal A2 A3
  constraint tangent L38 A4
  constraint tangent L39 A4
  constraint tangent L39 A5
  constraint tangent L40 A5
  constraint equal A4 A5
  constraint tangent L34 A6
  constraint tangent L35 A6
  constraint equal A4 A6
  constraint tangent L36 A7
  constraint tangent L35 A7
  constraint equal A4 A7
  constraint tangent L36 A8
  constraint tangent L37 A8
  constraint equal A4 A8
  constraint tangent L34 A9
  constraint tangent L37 A9
  constraint equal A4 A9
  measures "d992" distance of L0.start L0.end
  measures "d993" distance of L0.start L10.end
  measures "d997" distance of L0.start L15.end
  measures "d998" distance of L16.end L19.end
  measures "d999" distance of L19.end L20.end
  measures "d1000" distance of L19.end L22.end
  measures "d1001" distance of L9.end L24.end
  measures "d1002" distance of L25.end L28.end
  measures "d1003" distance of L28.end L29.end
  measures "d1004" diameter of A0
  measures "d1008" radius of A2
  measures "d1009" radius of A4
extrude "Extruir6" cut sketch "Boceto5" along normal blind -200 and the other way blind 50 contours L16 L19 L20 L21 L22 L23 | L25 L28 L29 L30 L31 L32 | L33 A0 | L33 A0
extrude "Extruir7" cut sketch "Boceto5" against normal blind 50 contours L16 L17 L23 L41 A3 | L16 L21 L22 L33 L39 L40 A3 A5 | L16 L19 L20 L21 L22 L23 | L17 L19 L20 L21 L23 L33 L38 L39 L41 A2 A4 | L26 L30 L31 L32 L33 L35 L36 L37 A7 A8 | L25 L26 L28 L32 L37 A9 | L25 L28 L29 L30 L31 L32 | L25 L29 L30 L33 L34 L35 A6 A9 | L33 A0 A1 | L33 A0 A1 | L33 A0 | L33 A0
sketch "Boceto6" plane through (0, 0, 0) normal (-1, 0, 0) x (0, -1, 0)
  line L0 (-800, 0) -> (0, 0)
  line L1 (0, 0) -> (0, 105)
  line L2 (0, 105) -> (-800, 105)
  line L3 (-800, 105) -> (-800, 0)
  line L4 (-800, 105) -> (0, 105)
  line L5 (-800, 0) -> (-800, 105)
  line L6 (-800, 0) -> (0, 0)
  line L7 (0, 0) -> (0, 105)
  line L8 (-500, 35) -> (-500, 15)
  line L9 (-493, 32) -> (-493, 18)
  line L10 (0, 105) -> (-800, 105)
  line L11 (-800, 0) -> (0, 0)
  line L12 (-800, 105) -> (-800, 0)
  circle A0 centre (-400, 25) radius 10
  line L13 (0, 0) -> (0, 105)
  line L14 (0, 50) -> (-800, 50)
  line L15 (-503, 8) -> (-657, 8)
  line L16 (0, 25) -> (0, 50)
  line L17 (0, 50) -> (-140, 50)
  line L18 (-660, 25) -> (-800, 25)
  line L19 (-500, 25) -> (-300, 25)
  line L20 (-660, 25) -> (-660, 35)
  line L21 (0, 0) -> (0, 105)
  line L22 (-140, 25) -> (0, 25)
  line L23 (-800, 0) -> (-660, 0)
  line L24 (-800, 0) -> (0, 0)
  arc A1 (-493, 32) -> (-503, 42) centre (-503, 32) ccw
  line L25 (-657, 42) -> (-503, 42)
  line L26 (-800, 105) -> (0, 105)
  arc A2 (-503, 8) -> (-493, 18) centre (-503, 18) ccw
  line L27 (-800, 0) -> (0, 0)
  line L28 (-140, 15) -> (-140, 35)
  line L29 (-800, 50) -> (-800, 0)
  line L30 (-140, 50) -> (-140, 25)
  arc A3 (-657, 42) -> (-667, 32) centre (-657, 32) ccw
  line L31 (-800, 25) -> (-800, 0)
  line L32 (-800, 15) -> (-800, 50)
  arc A4 (-667, 18) -> (-657, 8) centre (-657, 18) ccw
  line L33 (-800, 0) -> (-800, 105)
  line L34 (-300, 15) -> (-140, 15)
  circle A5 centre (-400, 25) radius 19
  line L35 (-299, 6) -> (-141, 6)
  arc A6 (-131, 34) -> (-141, 44) centre (-141, 34) ccw
  line L36 (-667, 18) -> (-667, 32)
  line L37 (-309, 34) -> (-309, 16)
  line L38 (-660, 0) -> (-660, 25)
  line L39 (-660, 35) -> (-500, 35)
  line L40 (-500, 15) -> (-660, 15)
  line L41 (-800, 50) -> (-800, 25)
  line L42 (0, 0) -> (0, 50)
  line L43 (-141, 44) -> (-299, 44)
  arc A7 (-299, 44) -> (-309, 34) centre (-299, 34) ccw
  line L44 (-140, 25) -> (-140, 35)
  line L45 (-140, 35) -> (-300, 35)
  line L46 (-300, 35) -> (-300, 15)
  line L47 (-660, 15) -> (-660, 35)
  line L48 (-800, 50) -> (-700, 50)
  arc A8 (-309, 16) -> (-299, 6) centre (-299, 16) ccw
  arc A9 (-141, 6) -> (-131, 16) centre (-141, 16) ccw
  line L49 (-131, 16) -> (-131, 34)
  point P0 (-800, 0)
  dimension "d1016" = 9
  dimension "d1017" = 800
  dimension "d1018" = 50
  dimension "d1019" = 140
  dimension "d1020" = 10
  dimension "d1021" = 160
  dimension "d1022" = 20
  dimension "d1023" = 140
  dimension "d1024" = 10
  dimension "d1025" = 160
  dimension "d1026" = 20
  dimension "d1027" = 7
  dimension "d1028" = 7
  dimension "d1029" = 7
  dimension "d1030" = 7
  dimension "d1031" = 10
  dimension "d1032" = 10
  dimension "d1033" = 9
  dimension "d1034" = 9
  dimension "d1035" = 9
  dimension "d1036" = 9
  constraint horizontal L24
  constraint vertical L42
  constraint horizontal L14
  constraint vertical L29
  constraint coincident P0 L0.start
  constraint midpoint L18.end L29
  constraint horizontal L48
  constraint vertical L32
  constraint horizontal L23
  constraint vertical L38
  constraint horizontal L18
  constraint vertical L31
  constraint perpendicular L14 L20
  constraint horizontal L39
  constraint vertical L8
  constraint horizontal L40
  constraint vertical L47
  constraint horizontal L17
  constraint vertical L30
  constraint horizontal L22
  constraint vertical L16
  constraint perpendicular L22 L44
  constraint horizontal L45
  constraint vertical L46
  constraint horizontal L34
  constraint vertical L28
  constraint midpoint L19.start L8
  constraint midpoint L19.end L46
  constraint perpendicular L19 L46
  constraint midpoint A0.centre L19
  constraint tangent L25 A3
  constraint tangent A3 L36
  constraint tangent L15 A4
  constraint tangent A4 L36
  constraint equal A3 A4
  constraint tangent A1 L25
  constraint tangent L9 A1
  constraint tangent L9 A2
  constraint tangent L15 A2
  constraint equal A1 A2
  constraint tangent L43 A7
  constraint tangent L37 A7
  constraint equal A1 A7
  constraint tangent L35 A8
  constraint tangent L37 A8
  constraint equal A1 A8
  constraint tangent L35 A9
  constraint tangent A9 L49
  constraint equal A1 A9
  constraint tangent A6 L43
  constraint tangent A6 L49
  constraint equal A1 A6
  measures "d1017" distance of L0.end P0
  measures "d1018" distance of L14.end P0
  measures "d1019" distance of L23.end P0
  measures "d1020" distance of L18.start L20.end
  measures "d1021" distance of L8.start L20.end
  measures "d1022" distance of L40.end L20.end
  measures "d1023" distance of L17.end L14.start
  measures "d1024" distance of L28.end L22.start
  measures "d1025" distance of L28.end L45.end
  measures "d1026" diameter of A0
  measures "d1027" distance of L25 L39
  measures "d1028" distance of L8 L9
  measures "d1029" distance of L15 L40
  measures "d1030" distance of L36 L47
  measures "d1031" radius of A3
  measures "d1032" radius of A1
  measures "d1033" distance of L43 L45
  measures "d1034" distance of L37 L46
  measures "d1035" distance of L34 L35
  measures "d1036" distance of L28 L49
extrude "Extruir8" cut sketch "Boceto6" along normal blind -200 and the other way blind 50 contours L8 L20 L38 L39 L40 L47 | L28 L30 L34 L44 L45 L46 | A0 L19 | A0 L19
extrude "Extruir9" cut sketch "Boceto6" against normal blind 50 contours L8 L9 L15 L19 A2 A4 L38 L40 | L18 A4 L36 L38 L47 | L8 L20 L38 L39 L40 L47 | L8 L9 L18 L19 L20 A1 L25 A3 L36 L39 L47 | L19 L22 L28 L34 L35 L37 L46 A8 A9 L49 | L22 L28 L30 A6 L44 L49 | L28 L30 L34 L44 L45 L46 | L19 L30 A6 L37 L43 A7 L45 L46 | A0 L19 A5 | A0 L19 A5 | A0 L19 | A0 L19
extrude "Extruir10" add 1 faces at (50, 554.3333, 12.6667) along direction (-1, 0, 0) blind 15
sketch "Boceto7" plane through (35, 0, 0) normal (-1, 0, 0) x (0, -1, 0)
  line L0 (-500, 35) -> (-500, 15)
  line L1 (-500, 15) -> (-660, 15)
  line L2 (-660, 15) -> (-660, 35)
  line L3 (-660, 35) -> (-500, 35)
  arc A0 (-503, 8) -> (-493, 18) centre (-503, 18) ccw
  line L4 (-493, 18) -> (-493, 32)
  arc A1 (-493, 32) -> (-503, 42) centre (-503, 32) ccw
  line L5 (-503, 42) -> (-657, 42)
  arc A2 (-657, 42) -> (-667, 32) centre (-657, 32) ccw
  line L6 (-667, 32) -> (-667, 18)
  arc A3 (-667, 18) -> (-657, 8) centre (-657, 18) ccw
  line L7 (-657, 8) -> (-503, 8)
  line L8 (-660, 35) -> (-500, 35)
  line L9 (-500, 35) -> (-500, 15)
  line L10 (-500, 15) -> (-660, 15)
  line L11 (-660, 15) -> (-660, 35)
  line L12 (-657, 42) -> (-503, 42)
  arc A4 (-493, 32) -> (-503, 42) centre (-503, 32) ccw
  arc A5 (-657, 42) -> (-667, 32) centre (-657, 32) ccw
  line L13 (-667, 18) -> (-667, 32)
  arc A6 (-667, 18) -> (-657, 8) centre (-657, 18) ccw
  line L14 (-503, 8) -> (-657, 8)
  arc A7 (-503, 8) -> (-493, 18) centre (-503, 18) ccw
  line L15 (-493, 32) -> (-493, 18)
  constraint horizontal L8
  constraint vertical L9
  constraint horizontal L10
  constraint vertical L11
  constraint coincident L0.end L1.start
  constraint coincident L2.end L3.start
sketch "Boceto8" plane through (35, 580, 25) normal (-1, 0, 0) x (0, -1, 0)
  line L0 (77, -17, 35) -> (-77, -17, 35)
  arc A0 through (77, -17, 35) (84.0711, -14.0711, 35) (87, -7, 35)
  line L1 (87, 7, 35) -> (87, -7, 35)
  arc A1 through (87, 7, 35) (84.0711, 14.0711, 35) (77, 17, 35)
  line L2 (-77, 17, 35) -> (77, 17, 35)
  arc A2 through (-77, 17, 35) (-84.0711, 14.0711, 35) (-87, 7, 35)
  line L3 (-87, -7, 35) -> (-87, 7, 35)
  arc A3 through (-87, -7, 35) (-84.0711, -14.0711, 35) (-77, -17, 35)
equation "d900 = 180 deg - 15 deg"
equation "d144 = 20.125 * 25.4 mm"
equation "d148 = 20.125 * 25.4 mm"
equation "d149 = 90 deg - 15 deg"
equation "d151 = 2.125 * 25.4 mm"
equation "d152 = 2.125 * 25.4 mm"
equation "d153 = 20.125 * 25.4 mm"
equation "d156 = 20.125 * 25.4 mm"
equation "d157 = 90 deg - 15 deg"
equation "d159 = 2.125 * 25.4 mm"
equation "d160 = 2.125 * 25.4 mm"
equation "d161 = 354.6390817817 * 0.5 mm"
equation "d162 = 2.75 * 25.4 mm"
equation "d164 = ( 2.75 * 25.4 ) * 1 mm"
equation "d165 = ( 15 * 0.5 ) * 1 mm"
equation "d166 = ( 15 * 0.5 ) * 1 mm"
equation "d167 = 354.6390817817 * 0.5 mm"
equation "d168 = 354.6390817817 * 0.5 mm"
equation "d169 = 354.6390817817 * 0.5 mm"
equation "d170 = 354.6390817817 * 0.5 mm"
equation "d179 = 25.4 * 2 mm"
equation "d219 = 90 mm + 15 mm"
equation "d387 = 90 mm + 15 mm"
equation "d391 = ( 15 / 2 ) * 1 mm"
equation "d392 = 27.5 mm + 15 mm"
equation "d395 = ( 15 / 2 ) * 1 mm"
equation "d401 = 90 mm + 15 mm"
equation "d404 = ( 15 / 2 ) * 1 mm"
equation "d405 = 27.5 mm + 15 mm"
equation "d408 = ( 15 / 2 ) * 1 mm"
equation "d416 = 90 mm + 15 mm"
equation "d420 = ( 15 / 2 ) * 1 mm"
equation "d421 = 27.5 mm + 15 mm"
equation "d424 = ( 15 / 2 ) * 1 mm"
equation "d430 = 90 mm + 15 mm"
equation "d433 = ( 15 / 2 ) * 1 mm"
equation "d434 = 27.5 mm + 15 mm"
equation "d437 = ( 15 / 2 ) * 1 mm"
equation "d443 = 90 mm + 15 mm"
equation "d446 = ( 15 / 2 ) * 1 mm"
equation "d447 = 27.5 mm + 15 mm"
equation "d450 = ( 15 / 2 ) * 1 mm"
equation "d458 = 90 mm + 15 mm"
equation "d462 = ( 15 / 2 ) * 1 mm"
equation "d463 = 27.5 mm + 15 mm"
equation "d466 = ( 15 / 2 ) * 1 mm"
equation "d472 = 90 mm + 15 mm"
equation "d475 = ( 15 / 2 ) * 1 mm"
equation "d476 = 27.5 mm + 15 mm"
equation "d479 = ( 15 / 2 ) * 1 mm"
equation "d488 = 90 mm + 15 mm"
equation "d492 = ( 15 / 2 ) * 1 mm"
equation "d493 = 27.5 mm + 15 mm"
equation "d496 = ( 15 / 2 ) * 1 mm"
equation "d501 = 90 mm + 15 mm"
equation "d504 = ( 15 / 2 ) * 1 mm"
equation "d505 = 27.5 mm + 15 mm"
equation "d508 = ( 15 / 2 ) * 1 mm"
equation "d250 = 180 deg - 15 deg"
equation "d277 = 180 deg - 15 deg"
equation "d304 = 180 deg - 15 deg"
equation "d333 = 90 mm + 15 mm"
equation "d342 = 90 mm + 15 mm"
equation "d351 = 90 mm + 15 mm"
equation "d367 = 20.125 * 25.4 mm"
equation "d369 = 20.125 * 25.4 mm"
equation "d370 = 90 deg - 15 deg"
equation "d372 = 2.125 * 25.4 mm"
equation "d373 = 2.125 * 25.4 mm"
equation "d374 = 354.6390817817 * 0.5 mm"
equation "d375 = ( 2.75 * 25.4 ) * 1 mm"
equation "d376 = ( 15 * 0.5 ) * 1 mm"
equation "d377 = ( 15 * 0.5 ) * 1 mm"
equation "d534 = 354.6390817817 * 0.5 mm"
equation "d535 = 354.6390817817 * 0.5 mm"
equation "d536 = 354.6390817817 * 0.5 mm"
equation "d537 = 354.6390817817 * 0.5 mm"
equation "d546 = 25.4 * 2 mm"
equation "d549 = 354.6390817817 * 0.5 mm"
equation "d550 = 354.6390817817 * 0.5 mm"